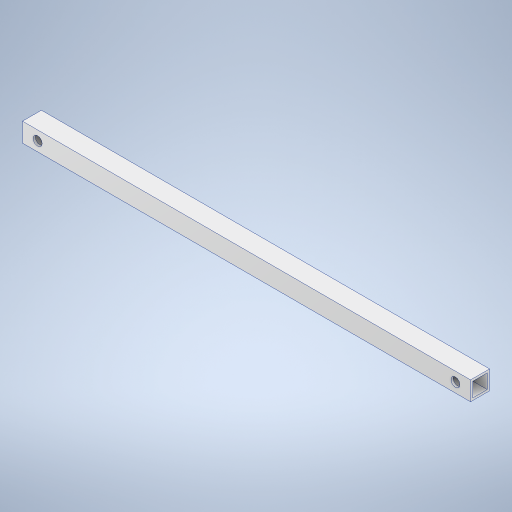
# Autodesk Inventor part: P001
Saved by Autodesk Inventor 2023 (Build 270158000, 158)
## iProperties
Created: 2022-08-29
Part Number: P001
Material: Aluminum 6061
Document SubType Name: Modeling
Designer: D.C. Eksteen
Density: 2.7 g/cm^3
Appearance: Aluminum - Flat
Author: D.C. Eksteen
Title: CONNECTING FRAME MEMBER
Autodesk Inventor part; units mm, degrees
ref_plane "YZ Plane" through (0, 0, 0) normal (1, 0, 0) x (0, 1, 0)
ref_plane "XZ Plane" through (0, 0, 0) normal (0, 1, 0) x (-1, 0, 0)
ref_plane "XY Plane" through (0, 0, 0) normal (0, 0, 1) x (1, 0, 0)
sketch "Sketch1" plane through (0, 0, 0) normal (1, 0, 0) x (0, 1, 0)
  line L0 (0, 0) -> (25, 0)
  line L1 (25, 0) -> (25, -25)
  line L2 (25, -25) -> (0, -25)
  line L3 (0, -25) -> (0, 0)
  line L4 (3, -3) -> (22, -3)
  line L5 (22, -3) -> (22, -22)
  line L6 (22, -22) -> (3, -22)
  line L7 (3, -22) -> (3, -3)
  dimension "d0" = 25
  dimension "d1" = 25
  dimension "d2" = 3
  constraints: 16 end point, 4 parallel, 2 perpendicular, 1 horizontal, 3 other
  measures "d0" distance of L1.end L2.end
  measures "d1" distance of L0.end L1.end
  measures "d2" distance between parallel lines of L3 L7
extrude "Extrusion1" add sketch "Sketch1" along normal blind 590
sketch "Sketch2" plane through (0, 0, 0) normal (0, 0, 1) x (1, 0, 0)
  line L0 (0, 25) -> (590, 25) projected
  line L1 (0, 0) -> (590, 0) projected
  point P0 (20, 12.5)
  point P1 (570, 12.5)
  point P2 (295, 25)
  dimension "d5" = 550
  dimension "d6" = 275
  dimension "d7" = 12.5
  dimension "d15" = 12.5
  constraints: 1 midpoint
  measures "d5" distance of point (570, 12.5) point (20, 12.5)
  measures "d6" horizontal distance of point (295, 25) point (20, 12.5)
  measures "d7" distance from line of L1 point (20, 12.5)
  measures "d15" distance from line of L1 point (570, 12.5)
hole "Hole1" at (20, 12.5, 0) at (570, 12.5, 0) direction (0, 0, -1) diameter 12 end through all
body "Solid1"
